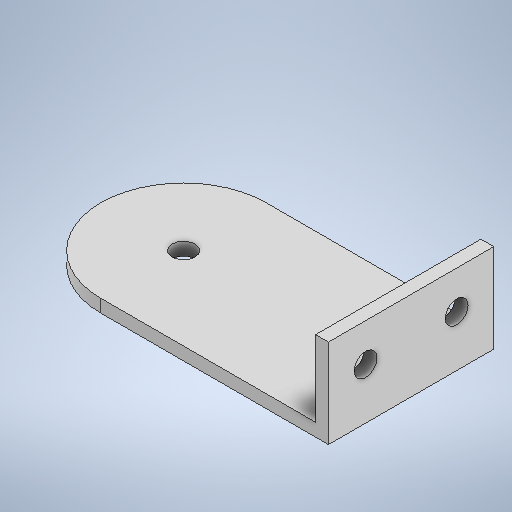
# Autodesk Inventor part: A3P3
Saved by Autodesk Inventor 2025.2 (Build 292293000, 293)
## iProperties
Created: 2025-05-22
Part Number: A3P3
Material: Generic
Document SubType Name: Sheet Metal
Designer: Admin
Density: 1 g/cm^3
Sheet Metal Rule: Default
Appearance: Default
Author: Admin
Autodesk Inventor part; units mm, degrees
ref_plane "YZ Plane" through (0, 0, 0) normal (1, 0, 0) x (0, 1, 0)
ref_plane "XZ Plane" through (0, 0, 0) normal (0, 1, 0) x (-1, 0, 0)
ref_plane "XY Plane" through (0, 0, 0) normal (0, 0, 1) x (1, 0, 0)
sketch "Sketch1" plane through (0, 0, 0) normal (0, 1, 0) x (-1, 0, 0)
  arc A0 (0, -10.9) -> (0, 10.9) centre (0, 0) ccw
  line L0 (0, -10.9) -> (-30, -10.9)
  line L1 (-30, -10.9) -> (-30, 10.9)
  line L2 (-30, 10.9) -> (0, 10.9)
  line L3 (0, 10.9) -> (0, -10.9) construction
  dimension "d2" = 10.9
  dimension "d3" = 30
  dimension "d4" = 30
  dimension "d5" = 21.8
  constraints: 8 end point, 2 point on circle, 1 centre point, 1 coincident, 1 parallel, 1 tangent, 1 vertical
  measures "d2" radius of A0
  measures "d3" distance of L1.end L2.end
  measures "d4" distance of L0.start L0.end
  measures "d5" distance of L0.end L1.end
extrude "Extrusion1" add sketch "Sketch1" along normal blind 1.7
sketch "Sketch2" plane through (0, 1.7, 0) normal (0, 1, 0) x (1, 0, 0)
  arc A0 (0, 10.9) -> (0, -10.9) centre (0, 0) ccw projected
  circle A1 centre (0, 0) radius 1.5
  dimension "d8" = 3
  constraints: 1 centre point, 1 coincident
  measures "d8" diameter of A1
extrude "Extrusion2" cut sketch "Sketch2" against normal blind 1.7
sketch "Sketch3" plane through (0, 1.7, 0) normal (0, 1, 0) x (1, 0, 0)
  line L0 (30, 10.9) -> (0, 10.9) projected
  line L1 (0, -10.9) -> (30, -10.9) projected
  line L2 (30, 10.9) -> (28.3, 10.9)
  line L3 (28.3, 10.9) -> (28.3, -10.9)
  line L4 (28.3, -10.9) -> (30, -10.9)
  line L5 (30, -10.9) -> (30, 10.9)
  point P0 (0, 0)
  dimension "d11" = 1.7
  constraints: 8 end point, 2 parallel, 1 horizontal, 1 perpendicular, 1 point on line
  measures "d11" distance of L4.end L3.end
extrude "Extrusion3" add sketch "Sketch3" along normal blind 10
sketch "Sketch4" plane through (28.3, 1.7, -10.9) normal (-1, 0, 0) x (0, 0, 1)
  circle A0 centre (4.9, 5) radius 1.5
  circle A1 centre (16.9, 5) radius 1.5
  line L0 (0, 10) -> (21.8, 10) projected
  line L1 (21.8, 0) -> (21.8, 10) projected
  point P0 (10.9, -1.7)
  dimension "d14" = 3
  dimension "d15" = 3
  dimension "d16" = 12
  dimension "d17" = 0
  dimension "d18" = 5
  dimension "d19" = 4.9
  constraints: 2 centre point
  measures "d14" diameter of A0
  measures "d15" diameter of A1
  measures "d16" distance of A1.centre A0.centre
  measures "d17" vertical distance of A1.centre A0.centre
  measures "d18" distance from line of L0 A1.centre
  measures "d19" distance from line of L1 A1.centre
extrude "Extrusion4" cut sketch "Sketch4" against normal blind 10
equation "\"BendRadius\" = Thickness"
equation "\"BendReliefWidth\" = Thickness"
equation "\"BendReliefDepth\" = 0.5 * Thickness"
equation "\"CornerReliefSize\" = 4 * Thickness"
equation "\"MinimumRemnant\" = 2 * Thickness"
equation "\"TransitionRadius\" = BendRadius"
equation "\"JacobiRadiusSize\" = BendRadius"
equation "\"GapSize\" = Thickness"
equation "\"Thickness\" = 3.048"
body "Solid1"
